fcf23c8c-fad9-4b38-a5c0-c952b8f856a3 (Autodesk Fusion 360 design; units mm, degrees)
Autodesk Fusion 360 part; units mm, degrees
note: some values were not read from the file. Set by a fixed rule: which sketch regions a step uses.
sketch "Sketch1" plane through (0, 0, 0) normal (0, 1, 0) x (1, 0, 0)
  circle A0 centre (0, 0) radius 9.525
  circle A1 centre (0, 0) radius 11.176
  circle A2 centre (0, 0) radius 7.9375
  circle A3 centre (0, 0) radius 8.9506
  arc A4 (11.1474, -0.7996) -> (-10.2436, -4.4688) centre (0, 0) ccw
  circle A5 centre (0, 0) radius 0.3969
  line L0 (0, 0) -> (11.176, 0) construction
  line L1 (0, 0) -> (-0.7801, -8.9165)
  line L2 (0, 0) -> (-1.5543, -8.8146)
  line L3 (0, 0) -> (-2.3166, -8.6456)
  line L4 (0, 0) -> (-3.0613, -8.4108)
  line L5 (0, 0) -> (-3.7827, -8.112)
  line L6 (0, 0) -> (-4.4753, -7.7514)
  line L7 (0, 0) -> (-5.1338, -7.3319)
  line L8 (-0.7801, -8.9165) -> (-0.002, -8.9846) construction
  line L9 (-1.5543, -8.8146) -> (-0.0158, -9.0859) construction
  line L10 (-2.3166, -8.6456) -> (-0.0532, -9.2521) construction
  line L11 (-3.0613, -8.4108) -> (-0.1254, -9.4794) construction
  line L12 (-3.7827, -8.112) -> (-0.2432, -9.7625) construction
  line L13 (-4.4753, -7.7514) -> (-0.4167, -10.0947) construction
  line L14 (-5.1338, -7.3319) -> (-0.655, -10.468) construction
  line L15 (0, 0) -> (-5.7533, -6.8565)
  line L16 (-5.7533, -6.8565) -> (-0.9666, -10.8731) construction
  line L17 (0, 0) -> (-6.329, -6.329)
  line L18 (-6.329, -6.329) -> (-1.3582, -11.2998) construction
  spline S0 degree 5 poles (-1.3582, -11.2998) (-1.3453, -11.2852) (-1.3195, -11.2561) (-1.2806, -11.213) (-1.2288, -11.1568) (-1.1644, -11.0882) (-1.1006, -11.0206) (-1.0382, -10.9535) (-0.9777, -10.8865) (-0.9193, -10.819) (-0.8632, -10.7509) (-0.8095, -10.6825) (-0.758, -10.6138) (-0.7085, -10.5451) (-0.6608, -10.4768) (-0.6147, -10.409) (-0.5702, -10.342) (-0.5272, -10.2757) (-0.4859, -10.2102) (-0.4463, -10.1454) (-0.4085, -10.0812) (-0.3726, -10.0177) (-0.3386, -9.9549) (-0.3064, -9.8929) (-0.276, -9.8319) (-0.2473, -9.772) (-0.2203, -9.7132) (-0.195, -9.6557) (-0.1715, -9.5995) (-0.1496, -9.5447) (-0.1294, -9.4913) (-0.1109, -9.4394) (-0.0941, -9.3891) (-0.0788, -9.3408) (-0.065, -9.2946) (-0.0526, -9.2506) (-0.0415, -9.2089) (-0.032, -9.1696) (-0.0239, -9.1325) (-0.0175, -9.0976) (-0.0125, -9.0654) (-0.0087, -9.0362) (-0.0056, -9.011) (-0.0029, -8.9903) (-0.0004, -8.9744) (0.0014, -8.963) (0.0019, -8.9568) (0.0013, -8.9533) (0.0005, -8.9514) (0, -8.9506) knots 0 0 0 0 0 0 0.022222 0.044444 0.066667 0.088889 0.111111 0.133333 0.155556 0.177778 0.2 0.222222 0.244444 0.266667 0.288889 0.311111 0.333333 0.355556 0.377778 0.4 0.422222 0.444444 0.466667 0.488889 0.511111 0.533333 0.555556 0.577778 0.6 0.622222 0.644444 0.666667 0.688889 0.711111 0.733333 0.755556 0.777778 0.8 0.822222 0.844444 0.866667 0.888889 0.911111 0.933333 0.955556 0.977778 1 1 1 1 1 1
  line L19 (-1.461, -11.4164) -> (-1.2555, -11.1832)
  line L20 (0.0374, -9.0097) -> (-0.0374, -8.8915)
  line L21 (-0.1419, -9.5239) -> (0, 0)
  line L22 (0, 0) -> (-0.8967, -6.107) construction
  line L23 (0, -8.9506) -> (0, 0) construction
  spline S1 degree 5 poles (0, -8.9506) (0, -8.8813) (0, -8.7556) (0, -8.6051) (0, -8.4669) (0, -8.3378) (0, -8.2184) (0, -8.0948) (0, -7.9932) (0, -7.9375) knots 0 0 0 0 0 0 0.2 0.4 0.6 0.8 1 1 1 1 1 1
  spline S2 degree 5 poles (-2.5731, -8.5727) (-2.5532, -8.5064) (-2.517, -8.386) (-2.4738, -8.2419) (-2.4341, -8.1095) (-2.3969, -7.9858) (-2.3626, -7.8715) (-2.3271, -7.7531) (-2.2979, -7.6557) (-2.2819, -7.6024) knots 0 0 0 0 0 0 0.2 0.4 0.6 0.8 1 1 1 1 1 1
  line L24 (0, -9.0389) -> (0, -8.8623)
  line L25 (0, -8.0085) -> (0, -7.8665)
  line L26 (-2.5985, -8.6573) -> (-2.5477, -8.4882)
  line L27 (-2.3023, -7.6704) -> (-2.2615, -7.5345)
  spline S3 degree 5 poles (-1.9476, -11.2133) (-1.9557, -11.1955) (-1.9721, -11.1602) (-1.9969, -11.1078) (-2.0304, -11.0391) (-2.0724, -10.9549) (-2.114, -10.8718) (-2.1545, -10.7896) (-2.1932, -10.708) (-2.2298, -10.6265) (-2.2639, -10.5453) (-2.2957, -10.4642) (-2.3252, -10.3836) (-2.3529, -10.3036) (-2.379, -10.2245) (-2.4036, -10.1463) (-2.427, -10.0693) (-2.4491, -9.9935) (-2.4699, -9.9189) (-2.4892, -9.8454) (-2.5069, -9.7731) (-2.523, -9.702) (-2.5376, -9.632) (-2.5506, -9.5634) (-2.5621, -9.4962) (-2.5724, -9.4306) (-2.5813, -9.3665) (-2.589, -9.3042) (-2.5955, -9.2436) (-2.6006, -9.1848) (-2.6046, -9.1278) (-2.6074, -9.0728) (-2.609, -9.0199) (-2.6098, -8.9692) (-2.6097, -8.9209) (-2.609, -8.8752) (-2.6076, -8.8321) (-2.6054, -8.7917) (-2.6025, -8.7538) (-2.5986, -8.7186) (-2.5941, -8.6863) (-2.5894, -8.6573) (-2.5851, -8.6322) (-2.5817, -8.6116) (-2.5795, -8.5957) (-2.5781, -8.5843) (-2.5767, -8.5781) (-2.5752, -8.5749) (-2.5738, -8.5734) (-2.5731, -8.5727) knots 0 0 0 0 0 0 0.022222 0.044444 0.066667 0.088889 0.111111 0.133333 0.155556 0.177778 0.2 0.222222 0.244444 0.266667 0.288889 0.311111 0.333333 0.355556 0.377778 0.4 0.422222 0.444444 0.466667 0.488889 0.511111 0.533333 0.555556 0.577778 0.6 0.622222 0.644444 0.666667 0.688889 0.711111 0.733333 0.755556 0.777778 0.8 0.822222 0.844444 0.866667 0.888889 0.911111 0.933333 0.955556 0.977778 1 1 1 1 1 1
  line L28 (-1.8827, -11.3545) -> (-2.0125, -11.072)
  line L29 (-2.6259, -8.6186) -> (-2.5203, -8.5269)
  point P0 (-0.1419, -9.5239)
  point P1 (0, -7.9375)
  point P2 (-2.2, -10.692)
  point P3 (-2.3819, -10.2144)
  point P4 (-2.5029, -9.7883)
  point P5 (-2.5736, -9.4203)
  point P6 (-2.6051, -9.1153)
  point P7 (-2.6089, -8.8768)
  point P8 (-2.5969, -8.7069)
  point P9 (-2.581, -8.6059)
  point P10 (-2.2819, -7.6024)
  dimension "d2" = 22.352
  dimension "id" = 15.875
  dimension "BaseDiameter" = 17.9011
  dimension "d1" = 0.7937
  dimension "d34" = 5
  dimension "d35" = 5
  dimension "d36" = 5
  dimension "d37" = 5
  dimension "d38" = 5
  dimension "d39" = 5
  dimension "d41" = 0.7811
  dimension "d42" = 1.5622
  dimension "d43" = 2.3433
  dimension "d44" = 3.1243
  dimension "d45" = 3.9054
  dimension "d46" = 4.6865
  dimension "d47" = 5.4676
  dimension "d48" = 5
  dimension "d49" = 6.2487
  dimension "d50" = 5
  dimension "d51" = 7.0298
  dimension "d55" = 7.5
  dimension "d60" = 5
  constraint coincident A0.centre A1.centre
  constraint concentric A0 A2
  constraint coincident A1 A4.end
  constraint horizontal L0
  constraint coincident A4 L0.end
  constraint coincident A3 S0.end
  constraint coincident A3 L1.end
  constraint coincident A3 L2.end
  constraint coincident A3 L3.end
  constraint coincident A3 L4.end
  constraint coincident A3 L5.end
  constraint coincident A3 L6.end
  constraint coincident A3 L7.end
  constraint vertical A0.centre S0.end
  constraint tangent A3 L8
  constraint tangent A3 L9
  constraint tangent A3 L10
  constraint tangent A3 L11
  constraint tangent A3 L12
  constraint tangent A3 L13
  constraint tangent A3 L14
  constraint coincident A3 L15.end
  constraint tangent A3 L16
  constraint coincident A3 L17.end
  constraint tangent A3 L18
  constraint midpoint L18.end L19
  constraint midpoint S0.end L20
  constraint coincident A0 P0
  constraint coincident S0 P0
  constraint coincident P0 L21.start
  constraint coincident L23 P1
  constraint coincident A2 P1
  constraint coincident P1 S1.end
  constraint midpoint S0.end L24
  constraint midpoint P1 L25
  constraint symmetric S0.end L22 S2.start
  constraint symmetric L8.end L22 P9
  constraint symmetric L9.end L22 P8
  constraint symmetric L10.end L22 P7
  constraint symmetric L11.end L22 P6
  constraint symmetric L12.end L22 P5
  constraint symmetric L13.end L22 P4
  constraint symmetric L14.end L22 P3
  constraint symmetric L16.end L22 P2
  constraint symmetric L18.end L22 S3.start
  constraint symmetric L19.start L22 L28.start
  constraint symmetric L19.end L22 L28.end
  constraint symmetric L20.start L22 L29.start
  constraint symmetric L20.end L22 L29.end
  constraint symmetric L22 P1 P10
  constraint symmetric L22 L24.start L26.start
  constraint symmetric L22 L24.end L26.end
  constraint symmetric L22 L25.start L27.start
  constraint symmetric L22 L25.end L27.end
  constraint vertical L24
  constraint vertical L25
  measures "d2" diameter of A1
  measures "id" diameter of A2
  measures "BaseDiameter" diameter of A3
  measures "d1" diameter of A5
  measures "d34" angle of L1 L2
  measures "d35" angle of L2 L3
  measures "d36" angle of L3 L4
  measures "d37" angle of L4 L5
  measures "d38" angle of L5 L6
  measures "d39" angle of L6 L7
  measures "d41" distance of L1.end L8.end
  measures "d42" distance of L2.end L9.end
  measures "d43" distance of L3.end L10.end
  measures "d44" distance of L4.end L11.end
  measures "d45" distance of L5.end L12.end
  measures "d46" distance of L6.end L13.end
  measures "d47" distance of L7.end L14.end
  measures "d48" angle of L7 L15
  measures "d49" distance of L15.end L16.end
  measures "d50" angle of L15 L17
  measures "d51" distance of L17.end L18.end
  measures "d55" angle of L21 L22
  measures "d60" angle of L1 L23
extrude "Extrude1" add sketch "Sketch1" along normal blind 304.8 contours A0 A1 S0 S3 | A3 S0 L21 | A0 A3 L21 S3 | A2 A3 L21 S1 L24 L25 | A2 A3 L1 L21 | A2 A3 L3 S2 L26 L27 | A2 A3 L1 L2 | A2 A3 L2 L3 makes body 1
pattern_circular "C-Pattern2" count 12 over 360 about axis through (0, 1.75, 0) along (0, 1, 0) of bodies 1 makes body 2 at (2.8081, 203.2, 7.4242) makes body 3 at (6.144, 203.2, 5.0255) makes body 4 at (7.8336, 203.2, 1.2802) makes body 5 at (7.3293, 203.2, -3.0471) makes body 6 at (5.0255, 203.2, -6.144) makes body 7 at (1.2802, 203.2, -7.8336) makes body 8 at (-2.8081, 203.2, -7.4242) makes body 9 at (-6.144, 203.2, -5.0255) makes body 10 at (-7.8336, 203.2, -1.2802) makes body 11 at (-7.4242, 203.2, 2.8081) makes body 12 at (-5.0255, 203.2, 6.144)
extrude "Extrude2" add sketch "Sketch1" along normal blind 304.8 contours A2 A5 L17 L21 | A2 A5 L1 L21 | A2 A5 L1 L2 | A2 A5 L3 L4 | A2 A5 L4 L5 | A2 A5 L2 L3 | A2 A5 L15 L17 | A2 A5 L5 L6 | A2 A5 L7 L15 | A2 A5 L6 L7 bodies 1 2 3 4 5 6 7 8 9 10 11 12
ref_plane "WorkPlane1" through (6.2747, 152.4, -0.8261) normal (0.130526, 0, 0.991445) x (0.991445, 0, -0.130526)
fillet "Fillet1" [suppressed]
mirror "Mirror3" [suppressed]
pattern_circular "C-Pattern1" [suppressed]
equation "d = 0.75 in"
equation "OutsideDiameter = d2"
equation "PitchDiameter = d"
equation "id = PitchDiameter - 2 * ( PitchDiameter / TeethNumber )"
equation "BaseDiameter = PitchDiameter * cos(20 deg)"
equation "Length = 12 in"
equation "t = 12"
equation "ShaftDiameter = d1"
equation "TeethNumber = t"
equation "Pitch = 32"
equation "d30 = ( 1.25 * ( PitchDiameter / TeethNumber ) ) - ( PitchDiameter / TeethNumber )"
equation "Basecircum = PI * PitchDiameter * cos(20 deg)"
equation "d41 = Basecircum * 5 / 360"
equation "d42 = Basecircum * 10 / 360"
equation "d43 = Basecircum * 15 / 360"
equation "d44 = Basecircum * 20 / 360"
equation "d45 = Basecircum * 25 / 360"
equation "d46 = Basecircum * 30 / 360"
equation "d47 = Basecircum * 35 / 360"
equation "d49 = Basecircum * 40 / 360"
equation "d51 = Basecircum * 45 / 360"
equation "d55 = ( 360 / ( 4 * TeethNumber ) ) * 1 deg"
